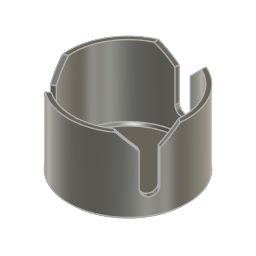
Cap For Magnetic Pickup tool (Autodesk Fusion 360 design; units mm, degrees)
Autodesk Fusion 360 part; units mm, degrees
sketch "Sketch1" plane through (0, 0, 0) normal (0, 0, 1) x (1, 0, 0)
  circle A0 centre (0, 0) radius 10.215
  circle A1 centre (0, 0) radius 11.015
  dimension "d22" = 20.43
  dimension "d23" = 0.8
  constraint coincident A0.centre A1.centre
  measures "d22" diameter of A0
extrude "Extrude1" add sketch "Sketch1" along normal blind 0.4 contours A0
extrude "Extrude2" add sketch "Sketch1" along normal blind 14
sketch "Sketch2" plane through (0, 0, 0) normal (0, 1, 0) x (1, 0, 0)
  line L0 (-11.015, -14) -> (11.015, -14)
  line L1 (-11.015, 0) -> (11.015, 0)
  line L2 (0, -14) -> (0, -4.9)
  line L3 (1.4, -14) -> (1.4, -4.9)
  arc A0 (1.4, -4.9) -> (-1.4, -4.9) centre (0, -4.9) ccw
  line L4 (-1.4, -4.9) -> (-1.4, -14)
  arc A1 (-1.4, -14) -> (1.4, -14) centre (0, -14) ccw
  line L5 (0, -14) -> (0, -4.9) construction
  dimension "d28" = 2.8
  dimension "d35" = 14
  dimension "d37" = 3.5
  constraint midpoint L0 L2.start
  constraint perpendicular L0 L2
  constraint tangent L3 A0
  constraint tangent A0 L4
  constraint parallel L3 L4
  constraint tangent L4 A1
  constraint tangent L3 A1
  constraint coincident L2.end A0.centre
  constraint perpendicular L0 L5
  constraint coincident L2.start A1.centre
  measures "d28" diameter of A0
  measures "d35" distance of L0.start L1
  measures "d37" distance of A0 origin
extrude "Extrude3" cut sketch "Sketch2" along normal through all contours L0 L3 A0 L4
pattern_circular "C-Pattern1" count 3 over 360 about axis through (0, 0, 1.75) along (0, 0, 1) of "Extrude3"
chamfer "Chamfer1" distance 0.4 angle 45 1 edges at (-9.5237, -3.6939, 0.4)
chamfer "Chamfer2" distance 0.4 angle 45 1 edges at (-10.2696, -3.9832, 0)
chamfer "Chamfer3" distance 3 angle 45 6 edges at (1.4, 10.5221, 14) (9.8124, -4.0486, 14) (8.4124, -6.4735, 14) (-1.4, 10.5221, 14) (-9.8124, -4.0486, 14) (-8.4124, -6.4735, 14)
equation "MagnetDiameter = 20.43 mm"
equation "WallThickness = 0.8 mm"
equation "FloorThickness = 0.4 mm"
equation "WallHeight = 14 mm"
equation "d22 = MagnetDiameter"
equation "d23 = WallThickness"
equation "d24 = FloorThickness"
equation "d26 = WallHeight"
equation "d28 = d35 * 0.2"
equation "d37 = d35 / 4"
named bodies: "Cap For Magnetic Pickup tool"
